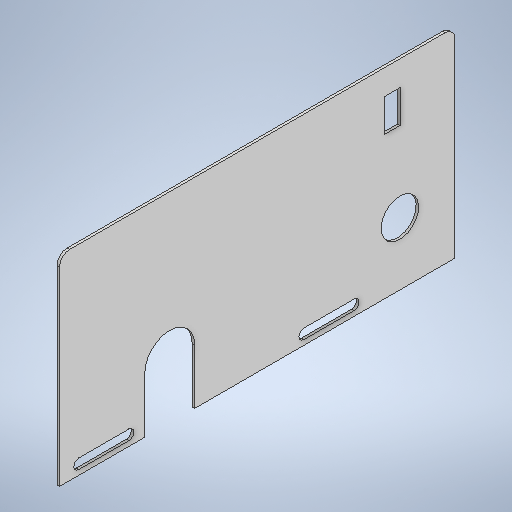
# Autodesk Inventor part: r2wall
Saved by Autodesk Inventor 2025.2 (Build 292293000, 293)
## iProperties
Created: 2026-05-19
Part Number: r2wall
Material: Generic
Document SubType Name: Modeling
Designer: AdminOS
Density: 1 g/cm^3
Appearance: Default
Author: AdminOS
Autodesk Inventor part; units mm, degrees
ref_plane "YZ Plane" through (0, 0, 0) normal (1, 0, 0) x (0, 1, 0)
ref_plane "XZ Plane" through (0, 0, 0) normal (0, 1, 0) x (-1, 0, 0)
ref_plane "XY Plane" through (0, 0, 0) normal (0, 0, 1) x (1, 0, 0)
sketch "Sketch1" plane through (0, 0, 0) normal (1, 0, 0) x (0, 1, 0)
  line L0 (0, 0) -> (380, 0)
  line L1 (400, -20) -> (400, -770)
  line L2 (380, -790) -> (0, -790)
  line L3 (0, -790) -> (0, 0)
  arc A0 (400, -20) -> (380, 0) centre (380, -20) ccw
  arc A1 (380, -790) -> (400, -770) centre (380, -770) ccw
  circle A2 centre (125, -680) radius 37.5
  line L4 (0, -170) -> (110, -170)
  line L5 (110, -270) -> (0, -270)
  line L6 (0, -270) -> (0, -170)
  arc A3 (110, -270) -> (110, -170) centre (110, -220) ccw
  line L7 (350, -680.5) -> (284.5, -680.5)
  line L8 (284.5, -680.5) -> (284.5, -650)
  line L9 (284.5, -650) -> (350, -650)
  line L10 (350, -650) -> (350, -680.5)
  line L11 (20, -588.3581) -> (20, -488.3581) construction
  line L12 (10, -588.3581) -> (10, -488.3581)
  line L13 (30, -488.3581) -> (30, -588.3581)
  arc A4 (10, -588.3581) -> (30, -588.3581) centre (20, -588.3581) ccw
  arc A5 (30, -488.3581) -> (10, -488.3581) centre (20, -488.3581) ccw
  arc A6 (10, -138.3581) -> (30, -138.3581) centre (20, -138.3581) ccw
  line L14 (20, -138.3581) -> (20, -38.3581) construction
  line L15 (10, -138.3581) -> (10, -38.3581)
  arc A7 (30, -38.3581) -> (10, -38.3581) centre (20, -38.3581) ccw
  line L16 (30, -38.3581) -> (30, -138.3581)
  point P0 (400, -790)
  point P1 (400, 0)
  point P2 (190, 0)
  point P3 (0, -270)
  point P4 (20, -538.3581)
  point P5 (30, -538.3581)
  point P6 (30, -88.3581)
  point P7 (20, -88.3581)
  dimension "d0" = 400
  dimension "d1" = 790
  dimension "d2" = 20
  dimension "d3" = 75
  dimension "d4" = 110
  dimension "d5" = 125
  dimension "d6" = 110
  dimension "d7" = 100
  dimension "d9" = 220
  dimension "d10" = 65.5
  dimension "d11" = 30.5
  dimension "d12" = 50
  dimension "d13" = 650
  dimension "d16" = 30
  dimension "d17" = 10
  dimension "d18" = 100
  dimension "d21" = 450
  constraints: 38 end point, 14 point on circle, 8 centre point, 8 tangent, 7 parallel, 5 point on line, 3 horizontal, 3 midpoint, 2 perpendicular, 2 vertical, 1 equal radius, 12 other
  measures "d0" distance of point (400, -790) L2.end
  measures "d1" distance of point (400, 0) point (400, -790)
  measures "d2" radius of A0
  measures "d3" diameter of A2
  measures "d4" distance from line of L2 A2.centre
  measures "d5" distance from line of L3 A2.centre
  measures "d6" distance of L5.start L5.end
  measures "d7" distance of L4.end L5.start
  measures "d9" distance from line of L0 A3.centre
  measures "d10" distance of L8.end L9.end
  measures "d11" distance of L7.end L8.end
  measures "d12" distance between parallel lines of L1 L10
  measures "d13" distance from line of point (190, 0) L9
  measures "d16" distance from line of L3 point (30, -538.358)
  measures "d17" radius of A5
  measures "d18" distance of L13.start L13.end
  measures "d21" distance of L11.end L14.end
extrude "Extrusion1" add sketch "Sketch1" along normal blind 5 contours L0 A0 L1 A1 L2 L3 L5 A3 L4
body "Solid1"
